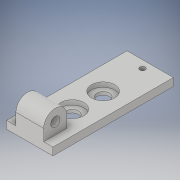
# Autodesk Inventor part: КВ33.044.601 - Опора держателя катка
Saved by Autodesk Inventor 2019 (Build 230136000, 136)
## iProperties
Created: 2019-07-22
Part Number: КВ33.044.601 - Опора держателя катка
Material: Типовые
Document SubType Name: Modeling
Designer: user
Density: 1 g/cm^3
Appearance: По умолчанию
Author: user
Autodesk Inventor part; units mm, degrees
ref_plane "YZ Plane" through (0, 0, 0) normal (1, 0, 0) x (0, 1, 0)
ref_plane "XZ Plane" through (0, 0, 0) normal (0, 1, 0) x (-1, 0, 0)
ref_plane "XY Plane" through (0, 0, 0) normal (0, 0, 1) x (1, 0, 0)
sketch "Эскиз1" plane through (0, 0, 0) normal (0, 1, 0) x (-1, 0, 0)
  line L0 (-14.9924, 37.5) -> (15.0076, 37.5)
  line L1 (15.0076, 37.5) -> (15.0076, -17.5)
  line L2 (15.0076, -17.5) -> (-14.9924, -17.5)
  line L3 (-14.9924, -17.5) -> (-14.9924, 37.5)
  circle A0 centre (0, -10) radius 4.1
  circle A1 centre (0, 10) radius 4.1
  line L4 (15.0076, -17.5) -> (-14.9924, -17.5)
  line L5 (-14.9924, -17.5) -> (-14.9924, -40.5)
  line L6 (-14.9924, -40.5) -> (15.0076, -40.5)
  line L7 (15.0076, -40.5) -> (15.0076, -17.5)
  point P0 (0, 0)
  dimension "d0" = 30
  dimension "d1" = 55
  dimension "d2" = 8.2
  dimension "d3" = 8.2
  dimension "d4" = 10
  dimension "d5" = 10
  dimension "d11" = 23
  constraints: 16 end point, 4 parallel, 2 centre point, 2 horizontal, 2 perpendicular
  measures "d0" distance of L1.end L2.end
  measures "d1" distance of L0.end L1.end
  measures "d2" diameter of A0
  measures "d3" diameter of A1
  measures "d4" distance of point (0, 0) A1.centre
  measures "d5" distance of A0.centre point (0, 0)
  measures "d11" distance of L5.end L4.end
extrude "Выдавливание1" add sketch "Эскиз1" along normal blind 5
sketch "Эскиз4" plane through (0, 5, 0) normal (0, 1, 0) x (1, 0, 0)
  line L0 (14.9924, -37.5) -> (-15.0076, -37.5) projected
  line L1 (-0.0076, -37.5) -> (-0.0076, -22.5)
  line L2 (8.9924, -37.5) -> (-9.0076, -37.5)
  line L3 (-9.0076, -37.5) -> (-9.0076, -22.5)
  line L4 (-9.0076, -22.5) -> (8.9924, -22.5)
  line L5 (8.9924, -22.5) -> (8.9924, -37.5)
  line L6 (8.9924, -37.5) -> (-9.0076, -22.5) construction
  line L7 (-9.0076, -37.5) -> (8.9924, -22.5) construction
  point P0 (0, 0)
  point P1 (-0.0076, -30)
  dimension "d19" = 15
  dimension "d20" = 18
  dimension "d21" = 15
  constraints: 14 end point, 4 midpoint, 2 parallel, 1 horizontal, 1 perpendicular, 1 vertical
  measures "d19" distance of L1.start L1.end
  measures "d20" distance of L3.end L4.end
  measures "d21" distance of L2.end L3.end
extrude "Выдавливание4" add sketch "Эскиз4" along normal blind 15
sketch "Эскиз5" plane through (8.9924, 5, 37.5) normal (1, 0, 0) x (0, 0, -1)
  line L0 (0, 15) -> (15, 15) projected
  line L1 (7.5, 15) -> (7.5, 0)
  line L2 (78, 0) -> (0, 0) projected
  circle A0 centre (7.5, 7.5) radius 3
  point P0 (37.5, -5)
  dimension "d24" = 6
  constraints: 2 end point, 2 midpoint, 1 centre point, 1 point on line, 1 vertical
  measures "d24" diameter of A0
extrude "Выдавливание5" cut sketch "Эскиз5" against normal blind 20
fillet "Сопряжение1" radius 7.5 2 edges at (-0.0076, 20, 22.5) (-0.0076, 20, 37.5)
sketch "Эскиз6" plane through (0, 5, 0) normal (0, 1, 0) x (1, 0, 0)
  line L0 (14.9924, 40.5) -> (-15.0076, 40.5) projected
  line L1 (-0.0076, 40.5) -> (-0.0076, 35.5)
  circle A0 centre (-0.0076, 35.5) radius 1.75
  point P0 (0, 0)
  dimension "d28" = 5
  dimension "d29" = 3.5
  constraints: 2 end point, 1 centre point, 1 coincident, 1 midpoint, 1 vertical
  measures "d28" distance of L1.start L1.end
  measures "d29" diameter of A0
extrude "Выдавливание6" cut sketch "Эскиз6" against normal blind 15
sketch "Эскиз7" plane through (0, 5, 0) normal (0, 1, 0) x (1, 0, 0)
  circle A0 centre (0, -10) radius 4.1 projected
  circle A1 centre (0, -10) radius 7.5
  circle A2 centre (0, 10) radius 4.1 projected
  circle A3 centre (0, 10) radius 7.5
  point P0 (0, 0)
  dimension "d32" = 15
  dimension "d33" = 15
  constraints: 2 centre point, 2 coincident
  measures "d32" diameter of A1
  measures "d33" diameter of A3
extrude "Выдавливание7" cut sketch "Эскиз7" against normal blind 3
